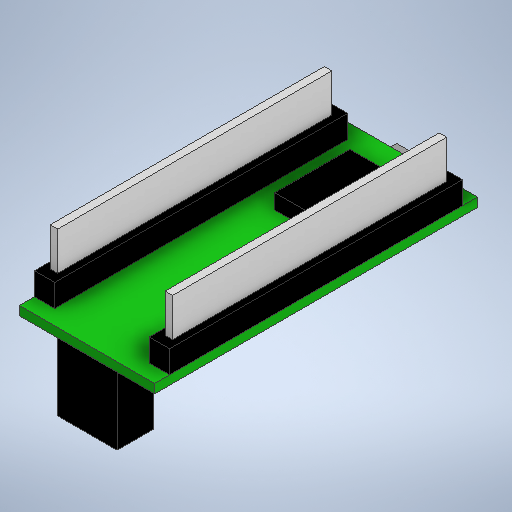
# Autodesk Inventor part: nano
Saved by Autodesk Inventor 2025.2 (Build 292293000, 293)
## iProperties
Created: 2025-04-04
Part Number: nano
Material: Generic
Document SubType Name: Modeling
Designer: joaki
Density: 1 g/cm^3
Appearance: Default
Author: joaki
Autodesk Inventor part; units mm, degrees
ref_plane "YZ Plane" through (0, 0, 0) normal (1, 0, 0) x (0, 1, 0)
ref_plane "XZ Plane" through (0, 0, 0) normal (0, 1, 0) x (-1, 0, 0)
ref_plane "XY Plane" through (0, 0, 0) normal (0, 0, 1) x (1, 0, 0)
sketch "Sketch1" plane through (0, 0, 0) normal (0, 1, 0) x (-1, 0, 0)
  line L0 (9.1437, 33.2437) -> (-8.8563, 33.2437)
  line L1 (-8.8563, 33.2437) -> (-8.8562, -9.7563)
  line L2 (-8.8562, -9.7563) -> (9.1438, -9.7563)
  line L3 (9.1438, -9.7563) -> (9.1437, 33.2437)
  point P0 (0, 0)
  dimension "d0" = 18
  dimension "d1" = 43
  constraints: 8 end point, 2 parallel, 1 horizontal, 1 perpendicular
  measures "d0" distance of L1.end L2.end
  measures "d1" distance of L2.end L0.start
extrude "Extrusion1" add sketch "Sketch1" along normal blind 1.2
sketch "Sketch2" plane through (0, 1.2, 0) normal (0, 1, 0) x (1, 0, 0)
  line L0 (-6.4427, -31.2437) -> (-9.1427, -31.2437)
  line L1 (-9.1427, -31.2437) -> (-9.1427, 7.7563)
  line L2 (-9.1427, 7.7563) -> (-6.4428, 7.7563)
  line L3 (-6.4428, 7.7563) -> (-6.4427, -31.2437)
  line L4 (-9.1438, 9.7563) -> (-9.1437, -33.2437) projected
  line L5 (8.8562, 9.7563) -> (-9.1438, 9.7563) projected
  line L6 (-9.1437, -33.2437) -> (8.8563, -33.2437) projected
  line L7 (-0.1437, -33.2437) -> (-0.1438, 9.7563)
  line L8 (6.1553, -31.2437) -> (8.8553, -31.2437)
  line L9 (8.8553, -31.2437) -> (8.8552, 7.7563)
  line L10 (8.8552, 7.7563) -> (6.1552, 7.7563)
  line L11 (6.1552, 7.7563) -> (6.1553, -31.2437)
  line L12 (8.8562, 9.7563) -> (8.8563, -33.2437)
  point P0 (0, 0)
  dimension "d4" = 0.001
  dimension "d5" = 2
  dimension "d6" = 2
  dimension "d7" = 2.7
  constraints: 20 end point, 4 symmetric about line, 2 midpoint, 2 parallel, 1 horizontal, 1 perpendicular
  measures "d4" distance between parallel lines of L4 L1
  measures "d5" distance between parallel lines of L5 L2
  measures "d6" distance between parallel lines of L6 L0
  measures "d7" distance between parallel lines of L1 L3
extrude "Extrusion2" add sketch "Sketch2" along normal blind 3 contours L0 L1 L2 L3 | L8 L11 L10 L9
sketch "Sketch3" plane through (0, 1.2, 0) normal (0, 1, 0) x (1, 0, 0)
  line L0 (2.8563, 4.7563) -> (-3.1437, 4.7563)
  line L1 (-3.1437, 4.7563) -> (-3.1437, -5.2437)
  line L2 (-3.1437, -5.2437) -> (2.8563, -5.2437)
  line L3 (2.8563, -5.2437) -> (2.8563, 4.7563)
  line L4 (8.8562, 9.7563) -> (-9.1438, 9.7563) projected
  line L5 (8.8563, -33.2437) -> (8.8562, 9.7563) projected
  line L6 (-9.1438, 9.7563) -> (-9.1437, -33.2437) projected
  point P0 (0, 0)
  dimension "d10" = 5
  dimension "d11" = 10
  dimension "d12" = 6
  dimension "d13" = 6
  constraints: 8 end point, 2 parallel, 1 horizontal, 1 perpendicular
  measures "d10" distance between parallel lines of L4 L0
  measures "d11" distance between parallel lines of L2 L0
  measures "d12" distance between parallel lines of L5 L3
  measures "d13" distance between parallel lines of L6 L1
extrude "Extrusion3" add sketch "Sketch3" along normal blind 2
sketch "Sketch4" plane through (0, 0, 0) normal (0, -1, 0) x (1, 0, 0)
  line L0 (-3.8938, -11.7563) -> (3.1062, -11.7563)
  line L1 (3.1062, -11.7563) -> (3.1062, -2.7563)
  line L2 (3.1062, -2.7563) -> (-3.8938, -2.7563)
  line L3 (-3.8938, -2.7563) -> (-3.8938, -11.7563)
  line L4 (-9.1438, -9.7563) -> (-9.1437, 33.2437) projected
  line L5 (8.8563, 33.2437) -> (8.8562, -9.7563) projected
  line L6 (8.8562, -9.7563) -> (-9.1438, -9.7563) projected
  point P0 (0, 0)
  dimension "d16" = 7
  dimension "d17" = 5.25
  dimension "d18" = 5.75
  dimension "d19" = 7
  dimension "d20" = 2
  constraints: 8 end point, 2 parallel, 1 horizontal, 1 perpendicular
  measures "d16" distance of L0.start L0.end
  measures "d17" distance between parallel lines of L4 L3
  measures "d18" distance between parallel lines of L5 L1
  measures "d19" distance between parallel lines of L6 L2
  measures "d20" distance between parallel lines of L6 L0
extrude "Extrusion4" add sketch "Sketch4" along normal blind 4
sketch "Sketch5" plane through (0, 0, 0) normal (0, -1, 0) x (1, 0, 0)
  line L0 (3.8563, 33.2427) -> (-4.1437, 33.2427)
  line L1 (-4.1437, 33.2427) -> (-4.1437, 28.3427)
  line L2 (-4.1437, 28.3427) -> (3.8563, 28.3427)
  line L3 (3.8563, 28.3427) -> (3.8563, 33.2427)
  line L4 (8.8563, 33.2437) -> (8.8562, -9.7563) projected
  line L5 (-9.1438, -9.7563) -> (-9.1437, 33.2437) projected
  line L6 (-9.1437, 33.2437) -> (8.8563, 33.2437) projected
  point P0 (0, 0)
  dimension "d23" = 5
  dimension "d24" = 5
  dimension "d25" = 0.001
  dimension "d26" = 4.9
  constraints: 8 end point, 2 parallel, 1 horizontal, 1 perpendicular
  measures "d23" distance between parallel lines of L4 L3
  measures "d24" distance between parallel lines of L5 L1
  measures "d25" distance between parallel lines of L6 L0
  measures "d26" distance between parallel lines of L0 L2
extrude "Extrusion5" add sketch "Sketch5" along normal blind 9
sketch "Sketch6" plane through (0, 4.2, 0) normal (0, 1, 0) x (1, 0, 0)
  line L0 (-8.2927, -29.9937) -> (-7.2927, -29.9937)
  line L1 (-7.2927, -29.9937) -> (-7.2928, 6.5063)
  line L2 (-7.2928, 6.5063) -> (-8.2927, 6.5063)
  line L3 (-8.2927, 6.5063) -> (-8.2927, -29.9937)
  line L4 (-9.1427, 7.7563) -> (-9.1427, -31.2437) projected
  line L5 (-6.4427, -31.2437) -> (-6.4428, 7.7563) projected
  line L6 (-9.1427, -31.2437) -> (-6.4427, -31.2437) projected
  line L7 (-6.4428, 7.7563) -> (-9.1427, 7.7563) projected
  line L8 (-9.1437, -33.2437) -> (8.8563, -33.2437) projected
  line L9 (-0.1437, -33.2437) -> (-0.1438, 9.7563)
  line L10 (8.8562, 9.7563) -> (-9.1438, 9.7563) projected
  line L11 (8.0053, -29.9937) -> (7.0053, -29.9937)
  line L12 (7.0053, -29.9937) -> (7.0052, 6.5063)
  line L13 (7.0052, 6.5063) -> (8.0052, 6.5063)
  line L14 (8.0052, 6.5063) -> (8.0053, -29.9937)
  line L15 (8.8552, 7.7563) -> (8.8553, -31.2437)
  line L16 (6.1553, -31.2437) -> (6.1552, 7.7563)
  line L17 (8.8553, -31.2437) -> (6.1553, -31.2437)
  line L18 (6.1552, 7.7563) -> (8.8552, 7.7563)
  point P0 (0, 0)
  point P1 (-7.7928, 6.5063)
  point P2 (-7.7927, -29.9937)
  point P3 (-7.7927, -31.2437)
  point P4 (-7.7927, 7.7563)
  point P5 (7.5052, 6.5063)
  point P6 (7.5053, -29.9937)
  point P7 (7.5053, -31.2437)
  point P8 (7.5052, 7.7563)
  dimension "d29" = 1
  dimension "d30" = 36.5
  dimension "d31" = 0.85
  dimension "d32" = 0.85
  dimension "d33" = 1.25
  dimension "d34" = 1.25
  constraints: 26 end point, 12 symmetric about line, 6 midpoint, 2 parallel, 1 horizontal, 1 perpendicular
  measures "d29" distance between parallel lines of L3 L1
  measures "d30" distance of point (-7.793, 6.506) point (-7.793, -29.994)
  measures "d31" distance between parallel lines of L4 L3
  measures "d32" distance between parallel lines of L5 L1
  measures "d33" distance of point (-7.793, -31.244) point (-7.793, -29.994)
  measures "d34" distance of point (-7.793, 7.756) point (-7.793, 6.506)
extrude "Extrusion6" add sketch "Sketch6" along normal blind 5.1 contours L3 L2 L1 L0 | L11 L12 L13 L14
body "Solid1"
